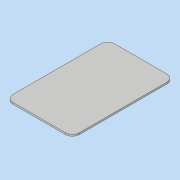
# Autodesk Inventor part: BatteryCaseSide3
Saved by Autodesk Inventor 2017 (Build 210142000, 142)
## iProperties
Created: 2018-02-15
Part Number: BatteryCaseSide3
Material: Generic
Document SubType Name: Modeling
Designer: Derek Wider
Density: 1 g/cm^3
Appearance: Default
Author: Derek Wider
Autodesk Inventor part; units mm, degrees
ref_plane "YZ Plane" through (0, 0, 0) normal (1, 0, 0) x (0, 1, 0)
ref_plane "XZ Plane" through (0, 0, 0) normal (0, 1, 0) x (-1, 0, 0)
ref_plane "XY Plane" through (0, 0, 0) normal (0, 0, 1) x (1, 0, 0)
sketch "Sketch1" plane through (0, 0, 0) normal (0, 1, 0) x (-1, 0, 0)
  line L0 (4.7625, 0) -> (53.0225, 0)
  line L1 (57.785, -4.7625) -> (57.785, -85.4075)
  line L2 (53.0225, -90.17) -> (4.7625, -90.17)
  line L3 (0, -85.4075) -> (0, -4.7625)
  arc A0 (57.785, -4.7625) -> (53.0225, 0) centre (53.0225, -4.7625) ccw
  arc A1 (4.7625, 0) -> (0, -4.7625) centre (4.7625, -4.7625) ccw
  arc A2 (0, -85.4075) -> (4.7625, -90.17) centre (4.7625, -85.4075) ccw
  arc A3 (53.0225, -90.17) -> (57.785, -85.4075) centre (53.0225, -85.4075) ccw
  line L4 (56.1975, -85.4075) -> (56.1975, -4.7625)
  arc A4 (56.1975, -4.7625) -> (53.0225, -1.5875) centre (53.0225, -4.7625) ccw
  line L5 (53.0225, -1.5875) -> (4.7625, -1.5875)
  arc A5 (4.7625, -1.5875) -> (1.5875, -4.7625) centre (4.7625, -4.7625) ccw
  line L6 (1.5875, -4.7625) -> (1.5875, -85.4075)
  arc A6 (1.5875, -85.4075) -> (4.7625, -88.5825) centre (4.7625, -85.4075) ccw
  line L7 (4.7625, -88.5825) -> (53.0225, -88.5825)
  arc A7 (53.0225, -88.5825) -> (56.1975, -85.4075) centre (53.0225, -85.4075) ccw
  line L8 (59.3725, -85.4075) -> (59.3725, -4.7625)
  arc A8 (59.3725, -4.7625) -> (53.0225, 1.5875) centre (53.0225, -4.7625) ccw
  line L9 (53.0225, 1.5875) -> (4.7625, 1.5875)
  arc A9 (4.7625, 1.5875) -> (-1.5875, -4.7625) centre (4.7625, -4.7625) ccw
  line L10 (-1.5875, -4.7625) -> (-1.5875, -85.4075)
  arc A10 (-1.5875, -85.4075) -> (4.7625, -91.7575) centre (4.7625, -85.4075) ccw
  line L11 (4.7625, -91.7575) -> (53.0225, -91.7575)
  arc A11 (53.0225, -91.7575) -> (59.3725, -85.4075) centre (53.0225, -85.4075) ccw
  line L12 (54.2925, -4.7625) -> (54.2925, -85.4075)
  arc A12 (53.0225, -86.6775) -> (54.2925, -85.4075) centre (53.0225, -85.4075) ccw
  line L13 (53.0225, -86.6775) -> (4.7625, -86.6775)
  arc A13 (3.4925, -85.4075) -> (4.7625, -86.6775) centre (4.7625, -85.4075) ccw
  line L14 (3.4925, -85.4075) -> (3.4925, -4.7625)
  arc A14 (4.7625, -3.4925) -> (3.4925, -4.7625) centre (4.7625, -4.7625) ccw
  line L15 (4.7625, -3.4925) -> (53.0225, -3.4925)
  arc A15 (54.2925, -4.7625) -> (53.0225, -3.4925) centre (53.0225, -4.7625) ccw
  line L16 (55.8165, -4.7625) -> (55.8165, -85.4075)
  arc A16 (53.0225, -88.2015) -> (55.8165, -85.4075) centre (53.0225, -85.4075) ccw
  line L17 (53.0225, -88.2015) -> (4.7625, -88.2015)
  arc A17 (1.9685, -85.4075) -> (4.7625, -88.2015) centre (4.7625, -85.4075) ccw
  line L18 (1.9685, -85.4075) -> (1.9685, -4.7625)
  arc A18 (4.7625, -1.9685) -> (1.9685, -4.7625) centre (4.7625, -4.7625) ccw
  line L19 (4.7625, -1.9685) -> (53.0225, -1.9685)
  arc A19 (55.8165, -4.7625) -> (53.0225, -1.9685) centre (53.0225, -4.7625) ccw
  point P0 (0, 0)
  point P1 (0, 0)
  point P2 (57.785, -90.17)
  point P3 (57.785, 0)
  point P4 (0, -90.17)
  dimension "d0" = 90.17
  dimension "d1" = 57.785
  dimension "d2" = 4.7625
  dimension "d3" = 1.5875
  dimension "d4" = 1.5875
  dimension "d5" = 1.905
  dimension "d6" = 0.381
  constraints: 40 end point, 40 point on circle, 20 centre point, 10 parallel, 8 point on line, 8 tangent, 5 perpendicular, 3 equal radius, 1 coincident, 1 horizontal, 28 other
  measures "d0" distance of point (57.785, 0) point (57.785, -90.17)
  measures "d1" distance of point (57.785, -90.17) point (0, -90.17)
  measures "d2" radius of A0
  measures "d3" distance between parallel lines of L1 L4
  measures "d4" distance between parallel lines of L1 L8
  measures "d5" distance between parallel lines of L4 L12
  measures "d6" distance between parallel lines of L4 L16
extrude "Extrusion1" add sketch "Sketch1" along normal blind 1.524 contours L0 A0 L1 A3 L2 A2 L3 A1 | A7 L7 A6 L6 A5 L5 A4 L4 | A11 L11 A10 L10 A9 L9 A8 L8 | L12 A12 L13 A13 L14 A14 L15 A15 | L16 A16 L17 A17 L18 A18 L19 A19
extrude "Extrusion2" add sketch "Sketch1" against normal blind 1.27 contours L16 A16 L17 A17 L18 A18 L19 A19
chamfer "Chamfer1" distance 0.762 angle 45 8 edges at (-28.8925, -1.27, -3.4925) (-3.8645, -1.27, -3.8645) (-3.4925, -1.27, -45.085) (-3.8645, -1.27, -86.3055) (-28.8925, -1.27, -86.6775) (-53.9205, -1.27, -86.3055) (-54.2925, -1.27, -45.085) (-53.9205, -1.27, -3.8645)
equation "\"d3\" = d4"
body "Solid1"
